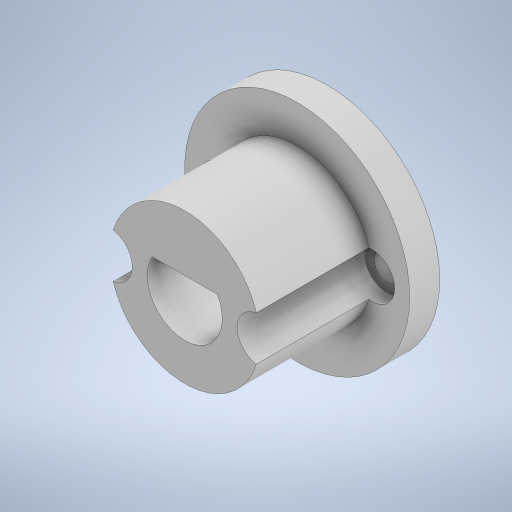
# Autodesk Inventor part: Motor-mount
Saved by Autodesk Inventor 2023 (Build 270158000, 158)
## iProperties
Created: 2023-01-18
Part Number: Motor-mount
Material: Generic
Document SubType Name: Modeling
Designer: caden
Density: 1 g/cm^3
Appearance: Default
Description: 3D Print
Author: caden
Autodesk Inventor part; units mm, degrees
ref_plane "YZ Plane" through (0, 0, 0) normal (1, 0, 0) x (0, 1, 0)
ref_plane "XZ Plane" through (0, 0, 0) normal (0, 1, 0) x (-1, 0, 0)
ref_plane "XY Plane" through (0, 0, 0) normal (0, 0, 1) x (1, 0, 0)
sketch "Sketch1" plane through (0, 0, 0) normal (0, 0, 1) x (1, 0, 0)
  circle A0 centre (0, 0) radius 15
  dimension "d0" = 30
  constraints: 1 centre point, 1 coincident
  measures "d0" diameter of A0
extrude "Extrusion1" add sketch "Sketch1" along normal blind 4
sketch "Sketch2" plane through (0, 0, 4) normal (0, 0, 1) x (1, 0, 0)
  circle A0 centre (0, 0) radius 10 construction
  line L0 (0, 0) -> (-11.9207, 0) construction
  point P0 (-10, 0)
  point P1 (10, 0)
  dimension "d10" = 20
  constraints: 2 end point, 2 point on circle, 1 centre point, 1 coincident, 1 horizontal, 1 point on line
  measures "d10" diameter of A0
hole "Hole1" at (-10, 0, 4) at (10, 0, 4) direction (0, 0, -1) diameter 3.5 end through all counterbore diameter 6 counterbore depth 2
sketch "Sketch4" plane through (0, 0, 4) normal (0, 0, 1) x (1, 0, 0)
  arc A0 (-4.3301, 2.5) -> (4.3301, 2.5) centre (0, 0) ccw
  line L0 (-4.3301, 2.5) -> (4.3301, 2.5)
  circle A1 centre (10, 0) radius 3 projected
  arc A2 (9.55, 2.9661) -> (9.55, -2.9661) centre (10, 0) ccw
  circle A3 centre (-10, 0) radius 3 projected
  arc A4 (-9.5586, -2.9382) -> (-9.5586, 2.9382) centre (-10, 0) ccw
  arc A5 (-9.5586, -2.9382) -> (9.55, -2.9661) centre (0, 0) ccw
  arc A6 (9.55, 2.9661) -> (-9.5586, 2.9382) centre (0, 0) ccw
  point P0 (9.55, 2.9661)
  point P1 (-9.55, 2.9661)
  point P2 (-9.55, -2.9661)
  dimension "d12" = 10
  dimension "d13" = 2.5
  dimension "d14" = 10
  dimension "d15" = 10
  constraints: 10 point on circle, 5 centre point, 4 coincident, 2 end point, 1 concentric, 1 horizontal
  measures "d12" diameter of A0
  measures "d13" distance from line of L0 point (0, 0)
  measures "d14" radius of A6
  measures "d15" radius of A5
extrude "Extrusion2" add sketch "Sketch4" along normal blind 15 contours A1 A5 A3 A6
equation "\"d15\" = d14"
body "Solid1"
